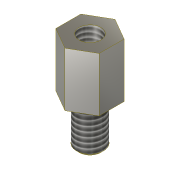
# Autodesk Inventor part: standoff (1466814)
Saved by Autodesk Inventor 2017 (Build 210142000, 142)
## iProperties
Part Number: standoff (1466814)
Material: Generisch
Document SubType Name: Modeling
Designer: ExCISS
Density: 1 g/cm^3
Appearance: Nickel
Author: ExCISS
Autodesk Inventor part; units mm, degrees
ref_plane "YZ Plane" through (0, 0, 0) normal (1, 0, 0) x (0, 1, 0)
ref_plane "XZ Plane" through (0, 0, 0) normal (0, 1, 0) x (-1, 0, 0)
ref_plane "XY Plane" through (0, 0, 0) normal (0, 0, 1) x (1, 0, 0)
sketch "Skizze1" plane through (0, 0, 0) normal (0, 0, 1) x (1, 0, 0)
  line L0 (-2, 0) -> (2, 0) construction
  line L1 (0, 2) -> (0, -2) construction
  line L2 (-2, 1.1547) -> (0, 2.3094)
  line L3 (0, 2.3094) -> (2, 1.1547)
  line L4 (2, 1.1547) -> (2, -1.1547)
  line L5 (2, -1.1547) -> (0, -2.3094)
  line L6 (0, -2.3094) -> (-2, -1.1547)
  line L7 (-2, -1.1547) -> (-2, 1.1547)
  point P0 (0, 0)
  point P1 (0, 0)
  point P2 (0, 0)
  dimension "d0" = 4
  dimension "d1" = 4
  dimension "d2" = 4
  constraints: 16 end point, 2 coincident, 2 midpoint, 1 horizontal, 1 perpendicular, 1 vertical, 13 other
  measures "d0" distance of L0.start L0.end
  measures "d1" distance of L1.start L1.end
  measures "d2" distance between parallel lines of L4 L7
extrude "Extrusion1" add sketch "Skizze1" along normal mid plane 5
sketch "Skizze3" plane through (0, 0, 2.5) normal (0, 0, 1) x (1, 0, 0)
  point P0 (0, 0)
  point P1 (0, 0)
  constraints: 1 coincident
hole "Bohrung1" at (0, 0, 2.5) direction (0, 0, -1) diameter 2.013 depth 3.5 tip angle 118 thread size "M2.5x0.45" class "6H" standard "ISO Metric profile"
sketch "Skizze4" plane through (0, 0, -2.5) normal (0, 0, -1) x (-1, 0, 0)
  circle A0 centre (0, 0) radius 1.25
  dimension "d17" = 2.5
  constraints: 1 centre point, 1 coincident
  measures "d17" diameter of A0
extrude "Extrusion3" add sketch "Skizze4" along normal blind 4
thread "Gewinde2" size "M2.5x0.45" class "6g" standard "ISO Metric profile" full length
chamfer "Fase1" distance 0.25 angle 45 1 edges at (1.25, 0, -6.5)
